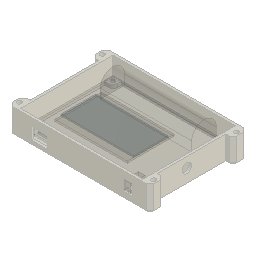
GNSS_Tracker_Enclosure (Autodesk Fusion 360 design; units mm, degrees)
Autodesk Fusion 360 part; units mm, degrees
note: some values were not read from the file. Set by a fixed rule: which sketch regions a step uses.
sketch "Sketch1" plane through (0, 0, 0) normal (0, 0, 1) x (1, 0, 0) in component "GNSS_PCB"
  line L0 (50.5, 37.875) -> (-50.5, 37.875)
  line L1 (-50.5, 37.875) -> (-50.5, -37.875)
  line L2 (-50.5, -37.875) -> (50.5, -37.875)
  line L3 (50.5, -37.875) -> (50.5, 37.875)
  line L4 (50.5, 37.875) -> (-50.5, -37.875) construction
  line L5 (-50.5, 37.875) -> (50.5, -37.875) construction
  line L6 (0, 37.875) -> (0, -37.875) construction
  line L7 (-50.5, 0) -> (50.5, 0) construction
  line L8 (-30.5, 8.425) -> (30.5, 8.425)
  line L9 (30.5, 8.425) -> (30.5, -31.075)
  line L10 (30.5, -31.075) -> (-30.5, -31.075)
  line L11 (-30.5, -31.075) -> (-30.5, 8.425)
  line L12 (-22, 1.425) -> (27.5, 1.425)
  line L13 (27.5, 1.425) -> (27.5, -24.075)
  line L14 (27.5, -24.075) -> (-22, -24.075)
  line L15 (-22, -24.075) -> (-22, 1.425)
  line L16 (-38.5, 35.825) -> (38.5, 35.825)
  line L17 (38.5, 35.825) -> (38.5, 15.175)
  line L18 (38.5, 15.175) -> (-38.5, 15.175)
  line L19 (-38.5, 15.175) -> (-38.5, 35.825)
  line L20 (-33.5, -37.875) -> (-33.5, 37.875) construction
  line L21 (40.5, -37.875) -> (40.5, 37.875) construction
  line L22 (-29, -30.475) -> (-38, -30.475)
  line L23 (-38, -30.475) -> (-38, -37.875)
  line L24 (-38, -37.875) -> (-29, -37.875)
  line L25 (-29, -37.875) -> (-29, -30.475)
  line L26 (-29, -30.475) -> (-38, -37.875) construction
  line L27 (-38, -30.475) -> (-29, -37.875) construction
  line L28 (43.25, -28.875) -> (37.75, -28.875)
  line L29 (37.75, -28.875) -> (37.75, -40.875)
  line L30 (37.75, -40.875) -> (43.25, -40.875)
  line L31 (43.25, -40.875) -> (43.25, -28.875)
  line L32 (43.25, -28.875) -> (37.75, -40.875) construction
  line L33 (37.75, -28.875) -> (43.25, -40.875) construction
  line L34 (50.5, -4) -> (-50.5, -4) construction
  line L35 (-30.5, 3.275) -> (30.5, 3.275)
  line L36 (30.5, 3.275) -> (30.5, -25.925)
  line L37 (30.5, -25.925) -> (-30.5, -25.925)
  line L38 (-30.5, -25.925) -> (-30.5, 3.275)
  point P0 (-48, 35.375)
  point P1 (48, 35.375)
  point P2 (48, -35.375)
  point P3 (-48, -35.375)
  point P4 (-33.5, -34.175)
  point P5 (40.5, -34.875)
  dimension "d6" = 75.75
  dimension "d8" = 101
  dimension "d9" = 2.5
  dimension "d10" = 2.5
  dimension "d19" = 61
  dimension "d20" = 39.5
  dimension "d21" = 30.5
  dimension "d22" = 8.425
  dimension "d23" = 49.5
  dimension "d24" = 25.5
  dimension "d25" = 7
  dimension "d26" = 8.5
  dimension "d30" = 77
  dimension "d31" = 20.65
  dimension "d32" = 38.5
  dimension "d35" = 35.825
  dimension "d38" = 17
  dimension "d39" = 10
  dimension "d43" = 9
  dimension "d44" = 7.4
  dimension "d45" = 7.4
  dimension "d49" = 5.5
  dimension "d50" = 12
  dimension "d51" = 9
  dimension "d74" = 61
  dimension "d75" = 29.2
  dimension "d76" = 5.15
  constraint horizontal L0
  constraint perpendicular L0 L1
  constraint parallel L0 L2
  constraint parallel L1 L3
  constraint coincident L4 origin
  constraint coincident L5 origin
  constraint midpoint L0 L6.start
  constraint midpoint L2 L6.end
  constraint midpoint L1 L7.start
  constraint midpoint L3 L7.end
  constraint symmetric P0 P1 L6
  constraint symmetric P1 P2 L7
  constraint symmetric P0 P3 L7
  constraint horizontal L8
  constraint vertical L9
  constraint horizontal L10
  constraint vertical L11
  constraint horizontal L12
  constraint vertical L13
  constraint horizontal L14
  constraint vertical L15
  constraint horizontal L16
  constraint vertical L17
  constraint horizontal L18
  constraint vertical L19
  constraint coincident L2 L20.start
  constraint coincident L0 L20.end
  constraint perpendicular L0 L20
  constraint coincident L2 L21.start
  constraint coincident L0 L21.end
  constraint perpendicular L0 L21
  constraint horizontal L22
  constraint perpendicular L22 L23
  constraint parallel L22 L24
  constraint parallel L23 L25
  constraint coincident L26 P4
  constraint coincident L27 P4
  constraint coincident L20 P4
  constraint horizontal L28
  constraint perpendicular L28 L29
  constraint parallel L28 L30
  constraint parallel L29 L31
  constraint coincident L32 P5
  constraint coincident L33 P5
  constraint coincident L21 P5
  constraint coincident L3 L34.start
  constraint coincident L1 L34.end
  constraint perpendicular L1 L34
  constraint horizontal L35
  constraint vertical L36
  constraint horizontal L37
  constraint vertical L38
  constraint coincident L11 L35.start
  measures "d6" distance of L0.end L1.end
  measures "d8" distance of L0.start L0.end
  measures "d9" distance of L0 P0
  measures "d10" distance of L1 P0
  measures "d19" distance of L8.start L8.end
  measures "d20" distance of L8.start L10.end
  measures "d21" distance of L6 L11
  measures "d22" distance of L7 L8
  measures "d23" distance of L12.start L12.end
  measures "d24" distance of L12.start L14.end
  measures "d25" distance of L8 L12
  measures "d26" distance of L11 L15
  measures "d30" distance of L16.start L16.end
  measures "d31" distance of L16.start L18.end
  measures "d32" distance of L6 L19
  measures "d35" distance of L7 L16
  measures "d38" distance of L1 L20
  measures "d39" distance of L3 L21
  measures "d43" distance of L23.end L24.end
  measures "d44" distance of L22.end L23.end
  measures "d45" distance of L2 L22
  measures "d49" distance of L29.end L30.end
  measures "d50" distance of L28.end L29.end
  measures "d51" distance of L2 L28
  measures "d74" distance of L35.start L35.end
  measures "d75" distance of L35.start L37.end
  measures "d76" distance of L8 L35
extrude "Extrude1" add sketch "Sketch1" along normal blind 1.6 contours L0 L1 L2 L3 L8 L9 L10 L11 L22 L23 L25 L28 L29 L31 L36 L38 | L2 L28 L29 L31 | L2 L10 L11 L22 L23 L24 L25 | L9 L10 L11 L22 L25 L37 | L10 L11 L22 L25 | L9 L11 L35 L36 L37 L38 | L8 L9 L11 L35 | L12 L13 L14 L15 | L16 L17 L18 L19 makes body 1 in component "GNSS_PCB"
sketch "Sketch2" plane through (0, 0, 1.6) normal (0, 0, 1) x (-1, 0, 0) in component "GNSS_PCB"
  line L0 (50.5, 37.875) -> (-50.5, 37.875)
  line L1 (-50.5, 37.875) -> (-50.5, -37.875)
  line L2 (-50.5, -37.875) -> (50.5, -37.875)
  line L3 (50.5, -37.875) -> (50.5, 37.875)
  line L4 (-37.75, 40.875) -> (-43.25, 40.875)
  line L5 (-37.75, 28.875) -> (-37.75, 40.875)
  line L6 (-43.25, 40.875) -> (-43.25, 28.875)
  line L7 (-40.5, 37.875) -> (-40.5, -37.875)
  line L8 (-38.5, -15.175) -> (38.5, -15.175)
  line L9 (-38.5, -35.825) -> (-38.5, -15.175)
  line L10 (38.5, -15.175) -> (38.5, -35.825)
  line L11 (38.5, -35.825) -> (-38.5, -35.825)
  line L12 (-43.25, 28.875) -> (-37.75, 28.875)
  point P0 (48, 35.375)
  point P1 (48, -35.375)
  point P2 (-48, -35.375)
  point P3 (-48, 35.375)
extrude "Extrude2" add sketch "Sketch2" along normal blind 18.5 contours L8 L9 L10 L11 bodies 1 in component "GNSS_PCB"
extrude "Extrude3" add sketch "Sketch2" along normal blind 7.5 contours L0 L5 L7 L12 | L0 L4 L5 L6 | L0 L6 L7 L12 bodies 1 in component "GNSS_PCB"
fillet "Fillet1" radius 10.325 1 edges at (0, 15.175, 20.1) on bodies 1 in component "GNSS_PCB"
fillet "Fillet2" radius 10.325 1 edges at (0, 35.825, 20.1) on bodies 1 in component "GNSS_PCB"
ref_plane "WorkPlane1" through (0, 0, 3.2) normal (0, 0, 1) x (-1, 0, 0) in component "GNSS_PCB"
sketch "Sketch3" plane through (0, 0, 3.2) normal (0, 0, 1) x (1, 0, 0) in component "GNSS_PCB"
  line L0 (-29, -30.475) -> (-38, -30.475)
  line L1 (-38, -30.475) -> (-38, -37.875)
  line L2 (-29, -37.875) -> (-29, -30.475)
  line L3 (-50.5, -37.875) -> (50.5, -37.875)
extrude "Extrude4" add sketch "Sketch3" along normal blind 1.6 separate body makes body 2 in component "GNSS_PCB"
ref_plane "WorkPlane2" through (0, 0, 12.6) normal (0, 0, 1) x (-1, 0, 0) in component "GNSS_PCB"
sketch "Sketch4" plane through (0, 0, 12.6) normal (0, 0, 1) x (1, 0, 0) in component "GNSS_PCB"
  line L0 (-30.5, 8.425) -> (30.5, 8.425)
  line L1 (-30.5, -31.075) -> (-30.5, 8.425)
  line L2 (30.5, 8.425) -> (30.5, -31.075)
  line L3 (30.5, -31.075) -> (-30.5, -31.075)
extrude "Extrude5" add sketch "Sketch4" along normal blind 1.6 separate body makes body 3 in component "GNSS_PCB"
sketch "Sketch5" plane through (0, 0, 14.2) normal (0, 0, 1) x (-1, 0, 0) in component "GNSS_PCB"
  line L0 (-30.5, 31.075) -> (-30.5, -8.425)
  line L1 (-30.5, -8.425) -> (30.5, -8.425)
  line L2 (30.5, -8.425) -> (30.5, 31.075)
  line L3 (30.5, 31.075) -> (-30.5, 31.075)
sketch "Sketch6" plane through (0, 0, 14.2) normal (0, 0, 1) x (-1, 0, 0) in component "GNSS_PCB"
  line L0 (30.5, -3.275) -> (-30.5, -3.275)
  line L1 (-30.5, 25.925) -> (30.5, 25.925)
  line L2 (30.5, 25.925) -> (30.5, -3.275)
  line L3 (-30.5, -3.275) -> (-30.5, 25.925)
extrude "Extrude6" add sketch "Sketch6" along normal blind 1.3 separate body makes body 4 in component "GNSS_PCB"
sketch "Sketch7" plane through (0, 0, 15.5) normal (0, 0, 1) x (-1, 0, 0) in component "GNSS_PCB"
  line L0 (-30.5, -3.275) -> (30.5, -3.275)
  line L1 (30.5, -3.275) -> (30.5, 25.925)
  line L2 (30.5, 25.925) -> (-30.5, 25.925)
  line L3 (-30.5, 25.925) -> (-30.5, -3.275)
  line L4 (-27.5, 24.075) -> (22, 24.075)
  line L5 (-27.5, -1.425) -> (-27.5, 24.075)
  line L6 (22, 24.075) -> (22, -1.425)
  line L7 (22, -1.425) -> (-27.5, -1.425)
hole "Hole1" at (-48, -35.375, 1.6) at (48, -35.375, 1.6) at (-48, 35.375, 1.6) at (48, 35.375, 1.6) direction (0, 0, -1) diameter 2.1 end through all bodies 1 in component "GNSS_PCB"
ref_plane "WorkPlane1" through (0, 0, -3) normal (0, 0, 1) x (1, 0, 0) in component "GNSS_Enclosure_Bottom"
sketch "Sketch1 (2)" plane through (0, 0, -3) normal (0, 0, 1) x (1, 0, 0) in component "GNSS_Enclosure_Bottom"
  line L0 (-50.5, -37.875) -> (50.5, -37.875)
  line L1 (50.5, -37.875) -> (50.5, 37.875)
  line L2 (50.5, 37.875) -> (-50.5, 37.875)
  line L3 (-50.5, 37.875) -> (-50.5, -37.875)
  line L4 (51.5, -38.875) -> (51.5, 38.875)
  line L5 (51.5, 38.875) -> (-51.5, 38.875)
  line L6 (-51.5, 38.875) -> (-51.5, -38.875)
  line L7 (-51.5, -38.875) -> (51.5, -38.875)
  line L8 (-53.5, -40.875) -> (53.5, -40.875)
  line L9 (53.5, -40.875) -> (53.5, 40.875)
  line L10 (53.5, 40.875) -> (-53.5, 40.875)
  line L11 (-53.5, 40.875) -> (-53.5, -40.875)
  circle A0 centre (-48, 35.375) radius 3.5
  circle A1 centre (48, 35.375) radius 3.5
  circle A2 centre (48, -35.375) radius 3.5
  circle A3 centre (-48, -35.375) radius 3.5
  line L12 (-44.5, 35.375) -> (-44.5, 38.875)
  line L13 (-48, 31.875) -> (-51.5, 31.875)
  line L14 (44.5, 35.375) -> (44.5, 38.875)
  line L15 (48, 31.875) -> (51.5, 31.875)
  line L16 (48, -31.875) -> (51.5, -31.875)
  line L17 (44.5, -35.375) -> (44.5, -38.875)
  line L18 (-48, -31.875) -> (-51.5, -31.875)
  line L19 (-44.5, -35.375) -> (-44.5, -38.875)
  point P0 (48, 35.375)
  point P1 (-48, 35.375)
  point P2 (-48, -35.375)
  point P3 (48, -35.375)
  dimension "d87" = 1
  dimension "d88" = 3
  constraint coincident P1 A0.centre
  constraint tangent L5 A0
  constraint coincident P0 A1.centre
  constraint tangent L5 A1
  constraint coincident P3 A2.centre
  constraint tangent L4 A2
  constraint coincident P2 A3.centre
  constraint tangent L7 A3
  constraint coincident A0 L12.start
  constraint coincident L5 L12.end
  constraint tangent A0 L12
  constraint perpendicular L5 L12
  constraint coincident A0 L13.start
  constraint coincident L6 L13.end
  constraint tangent A0 L13
  constraint perpendicular L6 L13
  constraint coincident A1 L14.start
  constraint coincident L5 L14.end
  constraint tangent A1 L14
  constraint perpendicular L5 L14
  constraint coincident A1 L15.start
  constraint coincident L4 L15.end
  constraint tangent A1 L15
  constraint perpendicular L4 L15
  constraint coincident A2 L16.start
  constraint coincident L4 L16.end
  constraint tangent A2 L16
  constraint perpendicular L4 L16
  constraint coincident A2 L17.start
  constraint coincident L7 L17.end
  constraint tangent A2 L17
  constraint perpendicular L7 L17
  constraint coincident A3 L18.start
  constraint coincident L6 L18.end
  constraint tangent A3 L18
  constraint perpendicular L6 L18
  constraint coincident A3 L19.start
  constraint coincident L7 L19.end
  constraint tangent A3 L19
  constraint perpendicular L7 L19
extrude "Extrude1'" add sketch "Sketch1 (2)" against normal blind 2 separate body contours L0 L3 A3 | L0 L3 L6 L7 A3 | L0 L3 A3 | L0 A3 | L3 A3 | L0 A3 L19 | L0 L7 A3 L19 | L3 L6 A3 L18 | L3 A3 L18 | L0 L1 L2 L3 A0 A1 A2 A3 L12 L13 L14 L15 L16 L17 L18 L19 | L0 L7 L17 L19 | L3 L6 L13 L18 | L0 A2 L17 | L0 L7 A2 L17 | L3 L6 A0 L13 | L3 A0 L13 | L0 L1 A2 | L0 A2 | L0 L1 L4 L7 A2 | L3 A0 | L2 L3 A0 | L2 L3 L5 L6 A0 | L0 L1 A2 | L1 A2 L16 | L2 L3 A0 | L2 A0 L12 | L1 A2 | L1 L4 A2 L16 | L1 L4 L15 L16 | L2 A0 | L2 L5 A0 L12 | L2 L5 L12 L14 | L1 A1 L15 | L1 L4 A1 L15 | L2 L5 A1 L14 | L2 A1 L14 | L1 L2 A1 | L1 A1 | L2 A1 | L1 L2 A1 | L1 L2 L4 L5 A1 | L8 L9 L10 L11 makes body 5 in component "GNSS_Enclosure_Bottom"
extrude "Extrude2'" add sketch "Sketch1 (2)" along normal up to surface (18.5 mm away) bodies 5 in component "GNSS_Enclosure_Bottom"
extrude "Extrude3'" add sketch "Sketch1 (2)" along normal blind 3 contours L0 L3 A3 | L0 L3 L6 L7 A3 | L0 L3 A3 | L0 A3 | L3 A3 | L0 A3 L19 | L0 L7 A3 L19 | L3 L6 A3 L18 | L3 A3 L18 | L0 A2 L17 | L0 L7 A2 L17 | L3 L6 A0 L13 | L3 A0 L13 | L0 L1 A2 | L0 A2 | L0 L1 L4 L7 A2 | L3 A0 | L2 L3 A0 | L2 L3 L5 L6 A0 | L1 A2 L16 | L2 A0 L12 | L1 A2 | L1 L4 A2 L16 | L2 A0 | L2 L5 A0 L12 | L1 A1 L15 | L1 L4 A1 L15 | L2 L5 A1 L14 | L2 A1 L14 | L1 L2 A1 | L1 A1 | L2 A1 | L1 L2 L4 L5 A1 picked at (48.5119, -35.209) picked at (-48.8502, 36.2083) picked at (47.5153, 35.9804) bodies 5 in component "GNSS_Enclosure_Bottom"
sketch "Sketch2 (2)" plane through (0, 0, 0) normal (0, 0, 1) x (-1, 0, 0) in component "GNSS_Enclosure_Bottom"
  line L0 (-50.5, -37.875) -> (-50.5, -37.8245)
  arc A0 (-50.5, -37.8245) -> (-50.4495, -37.875) centre (-48, -35.375) ccw
  line L1 (-50.4495, -37.875) -> (-50.5, -37.875)
  arc A1 (-44.5, -35.375) -> (-48, -31.875) centre (-48, -35.375) ccw
  line L2 (-48, -31.875) -> (-51.5, -31.875)
  line L3 (-51.5, -31.875) -> (-51.5, -38.875)
  line L4 (-51.5, -38.875) -> (-44.5, -38.875)
  line L5 (-44.5, -38.875) -> (-44.5, -35.375)
  point P0 (-48, 35.375)
  point P1 (48, 35.375)
  point P2 (48, -35.375)
  point P3 (-48, -35.375)
hole "Hole1'" at (48, -35.375, 0) at (-48, -35.375, 0) at (48, 35.375, 0) at (-48, 35.375, 0) direction (0, 0, -1) diameter 3.4 depth 3 tip angle 180 bodies 5 in component "GNSS_Enclosure_Bottom"
sketch "Sketch3 (2)" plane through (0, -40.875, 0) normal (0, -1, 0) x (1, 0, 0) in component "GNSS_Enclosure_Bottom"
  line L0 (-53.5, 15.5) -> (-53.5, -5)
  line L1 (-53.5, -5) -> (53.5, -5)
  line L2 (53.5, -5) -> (53.5, 15.5)
  line L3 (53.5, 15.5) -> (-53.5, 15.5)
  line L4 (-38, 3.2) -> (-29, 3.2)
  line L5 (-29, 3.2) -> (-29, 4.8)
  line L6 (-29, 4.8) -> (-38, 4.8)
  line L7 (-38, 4.8) -> (-38, 3.2)
  line L8 (37.75, 1.6) -> (43.25, 1.6)
  line L9 (43.25, 1.6) -> (43.25, 9.1)
  line L10 (43.25, 9.1) -> (37.75, 9.1)
  line L11 (37.75, 9.1) -> (37.75, 1.6)
  line L12 (36.75, 10.1) -> (36.75, 0.6)
  line L13 (36.75, 0.6) -> (44.25, 0.6)
  line L14 (44.25, 0.6) -> (44.25, 10.1)
  line L15 (44.25, 10.1) -> (36.75, 10.1)
  line L16 (-33.5, 4.8) -> (-33.5, 3.2) construction
  line L17 (-38, 4) -> (-29, 4) construction
  line L18 (-26.5, 9) -> (-40.5, 9)
  line L19 (-40.5, 9) -> (-40.5, -1)
  line L20 (-40.5, -1) -> (-26.5, -1)
  line L21 (-26.5, -1) -> (-26.5, 9)
  line L22 (-26.5, 9) -> (-40.5, -1) construction
  line L23 (-40.5, 9) -> (-26.5, -1) construction
  point P0 (-33.5, 4)
  dimension "d102" = 1
  dimension "d107" = 14
  dimension "d108" = 10
  constraint midpoint L6 L16.start
  constraint midpoint L4 L16.end
  constraint midpoint L7 L17.start
  constraint midpoint L5 L17.end
  constraint horizontal L18
  constraint perpendicular L18 L19
  constraint parallel L18 L20
  constraint parallel L19 L21
  constraint coincident L22 P0
  constraint coincident L23 P0
  constraint midpoint L17 P0
  measures "d107" distance of L19.end L20.end
  measures "d108" distance of L18.end L19.end
extrude "Extrude4'" cut sketch "Sketch3 (2)" against normal up to surface (2 mm away) contours L8 L9 L10 L11 | L12 L13 L14 L15 bodies 5 in component "GNSS_Enclosure_Bottom"
extrude "Extrude5'" cut sketch "Sketch3 (2)" against normal up to surface (2 mm away) contours L4 L5 L6 L7 | L18 L19 L20 L21 bodies 5 in component "GNSS_Enclosure_Bottom"
sketch "Sketch1 (3)" plane through (0, 0, 15.5) normal (0, 0, 1) x (-1, 0, 0) in component "GNSS_Enclosure_Top"
  line L0 (-51.5, -38.875) -> (-51.5, 38.875)
  line L1 (-51.5, 38.875) -> (51.5, 38.875)
  line L2 (51.5, 38.875) -> (51.5, -38.875)
  line L3 (51.5, -38.875) -> (-51.5, -38.875)
  line L4 (-53.5, -40.875) -> (53.5, -40.875)
  line L5 (53.5, -40.875) -> (53.5, 40.875)
  line L6 (53.5, 40.875) -> (-53.5, 40.875)
  line L7 (-53.5, 40.875) -> (-53.5, -40.875)
  line L8 (-38.5, -35.825) -> (-38.5, -15.175)
  line L9 (38.5, -35.825) -> (-38.5, -35.825)
  line L10 (-38.5, -15.175) -> (38.5, -15.175)
  line L11 (38.5, -15.175) -> (38.5, -35.825)
  line L12 (53.5, -40.875) -> (-53.5, -40.875)
  line L13 (53.5, 40.875) -> (53.5, -40.875)
  line L14 (-53.5, -40.875) -> (-53.5, 40.875)
  line L15 (-53.5, 40.875) -> (53.5, 40.875)
  line L16 (53.5, -10.125) -> (-53.5, -10.125)
  line L17 (-51.5, 38.875) -> (-51.5, -38.875)
  line L18 (-51.5, -38.875) -> (51.5, -38.875)
  line L19 (51.5, -38.875) -> (51.5, 38.875)
  dimension "d111" = 5.05
  dimension "d112" = 5.05
  constraint coincident L13 L16.start
  constraint coincident L14 L16.end
  constraint perpendicular L14 L16
  measures "d111" distance of L4 L9
  measures "d112" distance of L10 L16
extrude "Extrude1''" add sketch "Sketch1 (3)" along normal blind 2 separate body contours L0 L2 L3 L4 L5 L7 L12 L13 L14 L16 L17 L18 L19 | L0 L1 L2 L5 L6 L7 L13 L14 L15 L16 L17 L19 | L0 L1 L2 L16 L17 L19 makes body 6 in component "GNSS_Enclosure_Top"
sketch "Sketch2 (3)" plane through (0, 0, 17.5) normal (0, 0, 1) x (-1, 0, 0) in component "GNSS_Enclosure_Top"
  line L0 (51.5, -10.125) -> (51.5, -38.875)
  line L1 (51.5, -38.875) -> (-51.5, -38.875)
  line L2 (-51.5, -38.875) -> (-51.5, -10.125)
  line L3 (-51.5, -10.125) -> (51.5, -10.125)
  line L4 (-53.5, 40.875) -> (-53.5, -40.875)
  line L5 (-53.5, -40.875) -> (53.5, -40.875)
  line L6 (53.5, -40.875) -> (53.5, 40.875)
  line L7 (53.5, 40.875) -> (-53.5, 40.875)
  line L8 (-53.5, -8.125) -> (53.5, -8.125)
  dimension "d115" = 2
  constraint coincident L4 L8.start
  constraint coincident L6 L8.end
  constraint perpendicular L6 L8
  measures "d115" distance of L3 L8
sketch "Sketch3 (3)" plane through (53.5, 0, 0) normal (1, 0, 0) x (0, 1, 0) in component "GNSS_Enclosure_Top"
  line L0 (-40.875, 15.5) -> (40.875, 15.5)
  line L1 (40.875, 15.5) -> (40.875, 17.5)
  line L2 (40.875, 17.5) -> (-40.875, 17.5)
  line L3 (-40.875, 17.5) -> (-40.875, 15.5)
  arc A0 (35.825, 9.775) -> (15.175, 9.775) centre (25.5, 9.775) ccw
  line L4 (25.5, 20.1) -> (40.875, 20.1) construction
  line L5 (40.875, 20.1) -> (40.875, 17.5) construction
  line L6 (25.5, 22.1) -> (42.875, 22.1) construction
  line L7 (42.875, 22.1) -> (42.875, 17.5) construction
  constraint midpoint A0 L4.start
  constraint tangent A0 L4
  constraint perpendicular L1 L4
  constraint coincident L1.end L2.start
  constraint perpendicular L2 L5
extrude "Extrude2''" add sketch "Sketch2 (3)" along normal up to surface (4.6 mm away) contours L4 L5 L6 L8 bodies 6 in component "GNSS_Enclosure_Top"
sketch "Sketch4 (2)" plane through (0, 0, 22.1) normal (0, 0, 1) x (-1, 0, 0) in component "GNSS_Enclosure_Top"
  line L0 (51.5, -38.875) -> (-51.5, -38.875)
  line L1 (-51.5, -38.875) -> (-51.5, -10.125)
  line L2 (-51.5, -10.125) -> (51.5, -10.125)
  line L3 (51.5, -10.125) -> (51.5, -38.875)
  line L4 (-53.5, -8.125) -> (-53.5, -40.875)
  line L5 (-53.5, -40.875) -> (53.5, -40.875)
  line L6 (53.5, -40.875) -> (53.5, -8.125)
  line L7 (53.5, -8.125) -> (-53.5, -8.125)
extrude "Extrude3''" add sketch "Sketch4 (2)" along normal blind 2 contours L0 L1 L2 L3 | L4 L5 L6 L7 bodies 6 in component "GNSS_Enclosure_Top"
sketch "Sketch4 (3)" plane through (53.5, 0, 0) normal (1, 0, 0) x (0, 1, 0) in component "GNSS_Enclosure_Bottom"
  line L0 (-40.875, 15.5) -> (-40.875, -5)
  line L1 (-40.875, -5) -> (40.875, -5)
  line L2 (40.875, -5) -> (40.875, 15.5)
  line L3 (40.875, 15.5) -> (-40.875, 15.5)
  line L4 (-4, 0) -> (-4, 15.5) construction
  point P0 (-4, 0)
  point P1 (-4, 7.1)
  dimension "d124" = 7.1
  constraint coincident P0 L4.start
  constraint coincident L3 L4.end
  constraint perpendicular L3 L4
  constraint coincident L4 P1
  measures "d124" distance of P0 P1
hole "Hole2" at (53.5, -4, 7.1) direction (-1, 0, 0) diameter 8 depth 2 tip angle 180 bodies 5 in component "GNSS_Enclosure_Bottom"
sketch "Sketch5 (2)" plane through (0, 0, -5) normal (0, 0, -1) x (1, 0, 0) in component "GNSS_Enclosure_Bottom"
  line L0 (-53.5, 40.875) -> (-53.5, -40.875)
  line L1 (-53.5, -40.875) -> (53.5, -40.875)
  line L2 (53.5, -40.875) -> (53.5, 40.875)
  line L3 (53.5, 40.875) -> (-53.5, 40.875)
  line L4 (-53.5, 40.875) -> (-53.5, -40.875)
  line L5 (53.5, -40.875) -> (53.5, 40.875)
  line L6 (59.5, -40.875) -> (59.5, 40.875) construction
  line L7 (-59.5, 40.875) -> (-59.5, -40.875) construction
  line L8 (59.5, -40.875) -> (53.5, -40.875) construction
  line L9 (59.5, 40.875) -> (53.5, 40.875) construction
  line L10 (-59.5, -40.875) -> (-53.5, -40.875) construction
  line L11 (-59.5, 40.875) -> (-53.5, 40.875) construction
  line L12 (59.5, -28.875) -> (53.5, -28.875) construction
  line L13 (56.5, -40.875) -> (56.5, -28.875) construction
  line L14 (53.5, -40.875) -> (59.5, -40.875)
  line L15 (59.5, -28.875) -> (59.5, -40.875)
  line L16 (59.5, -28.875) -> (53.5, -28.875)
  line L17 (59.5, 28.875) -> (53.5, 28.875)
  line L18 (59.5, 28.875) -> (59.5, 40.875)
  line L19 (59.5, 40.875) -> (53.5, 40.875)
  line L20 (-59.5, -28.875) -> (-53.5, -28.875)
  line L21 (-59.5, 28.875) -> (-53.5, 28.875)
  line L22 (-53.5, -40.875) -> (-59.5, -40.875)
  line L23 (-59.5, -28.875) -> (-59.5, -40.875)
  line L24 (-59.5, 28.875) -> (-59.5, 40.875)
  line L25 (-59.5, 40.875) -> (-53.5, 40.875)
  line L26 (56.5, 28.875) -> (56.5, 40.875) construction
  line L27 (59.5, 34.875) -> (53.5, 34.875) construction
  line L28 (-56.5, -40.875) -> (-56.5, -28.875) construction
  line L29 (-56.5, 28.875) -> (-56.5, 40.875) construction
  point P0 (56.5, -34.875)
  point P1 (-56.5, -34.875)
  point P2 (-56.5, 34.875)
  point P3 (56.5, 34.875)
  dimension "d129" = 6
  dimension "d130" = 6
  dimension "d131" = 12
  dimension "d132" = 12
  dimension "d133" = 12
  dimension "d134" = 12
  constraint coincident L1.end L2.start
  constraint perpendicular L5 L8
  constraint coincident L2.end L3.start
  constraint perpendicular L5 L9
  constraint coincident L0.end L1.start
  constraint perpendicular L4 L10
  constraint coincident L0.start L3.end
  constraint perpendicular L4 L11
  constraint coincident L6 L12.start
  constraint coincident L2 L12.end
  constraint perpendicular L2 L12
  constraint midpoint L8 L13.start
  constraint midpoint L12 L13.end
  constraint midpoint L13 P0
  constraint coincident L6 L17.start
  constraint coincident L5 L17.end
  constraint perpendicular L5 L17
  constraint coincident L7 L20.start
  constraint coincident L0 L20.end
  constraint perpendicular L0 L20
  constraint coincident L7 L21.start
  constraint coincident L4 L21.end
  constraint perpendicular L4 L21
  constraint midpoint L17 L26.start
  constraint midpoint L9 L26.end
  constraint midpoint L18 L27.start
  constraint coincident L5 L27.end
  constraint perpendicular L5 L27
  constraint midpoint L10 L28.start
  constraint midpoint L20 L28.end
  constraint midpoint L21 L29.start
  constraint midpoint L25 L29.end
  constraint midpoint L28 P1
  constraint midpoint L29 P2
  constraint midpoint L26 P3
  measures "d131" distance of L8 L12
  measures "d132" distance of L9 L17
  measures "d133" distance of L10 L20
  measures "d134" distance of L11 L21
extrude "Extrude6'" add sketch "Sketch5 (2)" against normal up to surface (20.5 mm away) contours L0 L4 L21 L24 L25 | L2 L5 L17 L18 L19 | L0 L4 L20 L22 L23 | L2 L5 L14 L15 L16 bodies 5 in component "GNSS_Enclosure_Bottom"
chamfer "Chamfer1" distance 3 angle 45 8 edges at (59.5, -40.875, 5.25) (59.5, 40.875, 5.25) (59.5, 28.875, 5.25) (59.5, -28.875, 5.25) (-59.5, -40.875, 5.25) (-59.5, -28.875, 5.25) (-59.5, 28.875, 5.25) (-59.5, 40.875, 5.25) on bodies 5 in component "GNSS_Enclosure_Bottom"
sketch "Sketch6 (2)" plane through (0, 0, 15.5) normal (0, 0, 1) x (-1, 0, 0) in component "GNSS_Enclosure_Bottom"
  line L0 (-51.5, -38.875) -> (-51.5, 38.875)
  line L1 (-51.5, 38.875) -> (51.5, 38.875)
  line L2 (51.5, 38.875) -> (51.5, -38.875)
  line L3 (51.5, -38.875) -> (-51.5, -38.875)
  line L4 (56.5, -40.875) -> (59.5, -37.875)
  line L5 (59.5, -37.875) -> (59.5, -31.875)
  line L6 (59.5, -31.875) -> (56.5, -28.875)
  line L7 (56.5, -28.875) -> (53.5, -28.875)
  line L8 (53.5, -28.875) -> (53.5, 28.875)
  line L9 (53.5, 28.875) -> (56.5, 28.875)
  line L10 (56.5, 28.875) -> (59.5, 31.875)
  line L11 (59.5, 31.875) -> (59.5, 37.875)
  line L12 (59.5, 37.875) -> (56.5, 40.875)
  line L13 (56.5, 40.875) -> (-56.5, 40.875)
  line L14 (-56.5, 40.875) -> (-59.5, 37.875)
  line L15 (-59.5, 37.875) -> (-59.5, 31.875)
  line L16 (-59.5, 31.875) -> (-56.5, 28.875)
  line L17 (-56.5, 28.875) -> (-53.5, 28.875)
  line L18 (-53.5, 28.875) -> (-53.5, -28.875)
  line L19 (-53.5, -28.875) -> (-56.5, -28.875)
  line L20 (-56.5, -28.875) -> (-59.5, -31.875)
  line L21 (-59.5, -31.875) -> (-59.5, -37.875)
  line L22 (-59.5, -37.875) -> (-56.5, -40.875)
  line L23 (-56.5, -40.875) -> (56.5, -40.875)
  line L24 (-53.5, -28.875) -> (-53.5, -40.875)
  line L25 (53.5, -28.875) -> (53.5, -40.875)
  point P0 (-56.5, 34.875)
  point P1 (-56.5, -34.875)
  point P2 (56.5, -34.875)
  point P3 (56.5, 34.875)
  point P4 (-53.5, -40.875)
  point P5 (53.5, -40.875)
  constraint coincident L18.end L19.start
  constraint coincident P4 L24.end
  constraint coincident L7.end L8.start
  constraint coincident P5 L25.end
hole "Hole3" at (-56.5, -34.875, 15.5) at (-56.5, 34.875, 15.5) at (56.5, -34.875, 15.5) at (56.5, 34.875, 15.5) direction (0, 0, -1) diameter 3.4 depth 3 tip angle 180 bodies 5 in component "GNSS_Enclosure_Bottom"
chamfer "Chamfer2" distance 0.2 distance2 3 8 edges at (-58.085, 35.4897, 15.5) (54.915, 35.4897, 15.5) (-49.585, 35.9897, 0) (-58.085, -34.2603, 15.5) (54.915, -34.2603, 15.5) (46.415, 35.9897, 0) (46.415, -34.7603, 0) (-49.585, -34.7603, 0) measured on face at (54.557, -38.703, 15.5) measured on face at (54.557, -38.703, 15.5) measured on face at (-45.1759, 36.825, 0) measured on face at (54.557, -38.703, 15.5) measured on face at (54.557, -38.703, 15.5) measured on face at (45.1759, 36.825, 0) measured on face at (45.1759, -36.825, 0) measured on face at (-50.8984, -35.3327, 0) on bodies 5 in component "GNSS_Enclosure_Bottom"
sketch "Sketch5 (3)" plane through (0, 0, 15.5) normal (0, 0, -1) x (1, 0, 0) in component "GNSS_Enclosure_Top"
  line L0 (-51.5, -38.875) -> (-51.5, -10.125)
  line L1 (-51.5, -10.125) -> (51.5, -10.125)
  line L2 (51.5, -10.125) -> (51.5, -38.875)
  line L3 (51.5, -38.875) -> (-51.5, -38.875)
  line L4 (53.5, -40.875) -> (53.5, 40.875)
  line L5 (53.5, 40.875) -> (-53.5, 40.875)
  line L6 (-53.5, 40.875) -> (-53.5, -40.875)
  line L7 (-53.5, -40.875) -> (53.5, -40.875)
  circle A0 centre (-56.5, 34.875) radius 1.9
  circle A1 centre (-56.5, -34.875) radius 1.9
  line L8 (51.5, -38.875) -> (51.5, 38.875)
  line L9 (51.5, 38.875) -> (-51.5, 38.875)
  line L10 (-51.5, 38.875) -> (-51.5, -38.875)
  line L11 (-51.5, -38.875) -> (51.5, -38.875)
  line L12 (-56.5, -40.875) -> (-59.5, -37.875)
  line L13 (-59.5, -37.875) -> (-59.5, -31.875)
  line L14 (-59.5, -31.875) -> (-56.5, -28.875)
  line L15 (-56.5, -28.875) -> (-53.5, -28.875)
  line L16 (-53.5, -28.875) -> (-53.5, 28.875)
  line L17 (-53.5, 28.875) -> (-56.5, 28.875)
  line L18 (-56.5, 28.875) -> (-59.5, 31.875)
  line L19 (-59.5, 31.875) -> (-59.5, 37.875)
  line L20 (-59.5, 37.875) -> (-56.5, 40.875)
  line L21 (-56.5, 40.875) -> (56.5, 40.875)
  line L22 (56.5, 40.875) -> (59.5, 37.875)
  line L23 (59.5, 37.875) -> (59.5, 31.875)
  line L24 (59.5, 31.875) -> (56.5, 28.875)
  line L25 (56.5, 28.875) -> (53.5, 28.875)
  line L26 (53.5, 28.875) -> (53.5, -28.875)
  line L27 (53.5, -28.875) -> (56.5, -28.875)
  line L28 (56.5, -28.875) -> (59.5, -31.875)
  line L29 (59.5, -31.875) -> (59.5, -37.875)
  line L30 (59.5, -37.875) -> (56.5, -40.875)
  line L31 (56.5, -40.875) -> (-56.5, -40.875)
  circle A2 centre (56.5, -34.875) radius 1.9
  circle A3 centre (56.5, 34.875) radius 1.9
extrude "Extrude4''" add sketch "Sketch5 (3)" against normal up to surface (2 mm away) contours L4 L21 L22 L23 L24 L25 | L6 L17 L18 L19 L20 L21 | A0 | A3 bodies 6 in component "GNSS_Enclosure_Top"
extrude "Extrude5''" add sketch "Sketch6 (2)" along normal up to surface (8.6 mm away) contours L4 L5 L6 L7 L23 L25 | L19 L20 L21 L22 L23 L24 bodies 6 in component "GNSS_Enclosure_Top"
sketch "Sketch6 (3)" plane through (0, 0, 15.5) normal (0, 0, 1) x (1, 0, 0) in component "GNSS_Enclosure_Top"
sketch "Sketch7 (2)" plane through (0, 0, 17.5) normal (0, 0, 1) x (-1, 0, 0) in component "GNSS_Enclosure_Top"
  line L0 (-53.5, -8.125) -> (53.5, -8.125)
  line L1 (53.5, -8.125) -> (53.5, 28.875)
  line L2 (53.5, 28.875) -> (56.5, 28.875)
  line L3 (56.5, 28.875) -> (59.5, 31.875)
  line L4 (59.5, 31.875) -> (59.5, 37.875)
  line L5 (59.5, 37.875) -> (56.5, 40.875)
  line L6 (56.5, 40.875) -> (-56.5, 40.875)
  line L7 (-56.5, 40.875) -> (-59.5, 37.875)
  line L8 (-59.5, 37.875) -> (-59.5, 31.875)
  line L9 (-59.5, 31.875) -> (-56.5, 28.875)
  line L10 (-56.5, 28.875) -> (-53.5, 28.875)
  line L11 (-53.5, 28.875) -> (-53.5, -8.125)
  point P0 (56.5, 34.875)
  point P1 (-56.5, 34.875)
sketch "Sketch8" plane through (0, 0, 24.1) normal (0, 0, 1) x (-1, 0, 0) in component "GNSS_Enclosure_Top"
  line L0 (53.5, -8.125) -> (-53.5, -8.125)
  line L1 (-53.5, -8.125) -> (-53.5, -28.875)
  line L2 (-53.5, -28.875) -> (-56.5, -28.875)
  line L3 (-56.5, -28.875) -> (-59.5, -31.875)
  line L4 (-59.5, -31.875) -> (-59.5, -37.875)
  line L5 (-59.5, -37.875) -> (-56.5, -40.875)
  line L6 (-56.5, -40.875) -> (56.5, -40.875)
  line L7 (56.5, -40.875) -> (59.5, -37.875)
  line L8 (59.5, -37.875) -> (59.5, -31.875)
  line L9 (59.5, -31.875) -> (56.5, -28.875)
  line L10 (56.5, -28.875) -> (53.5, -28.875)
  line L11 (53.5, -28.875) -> (53.5, -8.125)
  point P0 (56.5, -34.875)
  point P1 (-56.5, -34.875)
hole "Hole1''" at (-56.5, 34.875, 24.1) at (56.5, 34.875, 24.1) direction (0, 0, -1) diameter 2.3 depth 8.6 tip angle 180 counterbore diameter 4 counterbore depth 2 bodies 6 in component "GNSS_Enclosure_Top"
hole "Hole2'" at (-56.5, -34.875, 17.5) at (56.5, -34.875, 17.5) direction (0, 0, -1) diameter 2.3 depth 2 tip angle 180 counterbore diameter 4 counterbore depth 1 bodies 6 in component "GNSS_Enclosure_Top"
sketch "Sketch9" plane through (0, 0, 17.5) normal (0, 0, 1) x (-1, 0, 0) in component "GNSS_Enclosure_Top"
  circle A0 centre (56.5, 34.875) radius 2
  circle A1 centre (-56.5, 34.875) radius 2
  line L0 (-53.5, -8.125) -> (53.5, -8.125)
  line L1 (53.5, -8.125) -> (53.5, 28.875)
  line L2 (53.5, 28.875) -> (56.5, 28.875)
  line L3 (56.5, 28.875) -> (59.5, 31.875)
  line L4 (59.5, 31.875) -> (59.5, 37.875)
  line L5 (59.5, 37.875) -> (56.5, 40.875)
  line L6 (56.5, 40.875) -> (-56.5, 40.875)
  line L7 (-56.5, 40.875) -> (-59.5, 37.875)
  line L8 (-59.5, 37.875) -> (-59.5, 31.875)
  line L9 (-59.5, 31.875) -> (-56.5, 28.875)
  line L10 (-56.5, 28.875) -> (-53.5, 28.875)
  line L11 (-53.5, 28.875) -> (-53.5, -8.125)
  line L12 (22, -1.425) -> (-27.5, -1.425)
  line L13 (22, 24.075) -> (22, -1.425)
  line L14 (-27.5, 24.075) -> (22, 24.075)
  line L15 (-27.5, -1.425) -> (-27.5, 24.075)
extrude "Extrude6''" cut sketch "Sketch9" against normal up to surface (2 mm away) contours L12 L13 L14 L15 bodies 6 in component "GNSS_Enclosure_Top"
chamfer "Chamfer1'" distance 2 angle 45 4 edges at (2.75, 1.425, 17.5) (27.5, -11.325, 17.5) (2.75, -24.075, 17.5) (-22, -11.325, 17.5) on bodies 6 in component "GNSS_Enclosure_Top"
chamfer "Chamfer2'" distance 1 angle 45 25 edges at (59.5, -34.875, 17.5) (58, -30.375, 17.5) (55, -28.875, 17.5) (53.5, -10.375, 17.5) (58, -39.375, 17.5) (0, -40.875, 17.5) (-58, -39.375, 17.5) (-59.5, -34.875, 17.5) (-58, -30.375, 17.5) (-55, -28.875, 17.5) (-53.5, -10.375, 17.5) (-53.5, 8.125, 20.8) (-53.5, 18.5, 24.1) (0, 8.125, 24.1) (-55, 28.875, 24.1) (-58, 30.375, 24.1) (-59.5, 34.875, 24.1) (-58, 39.375, 24.1) (0, 40.875, 24.1) (58, 39.375, 24.1) (59.5, 34.875, 24.1) (58, 30.375, 24.1) (55, 28.875, 24.1) (53.5, 18.5, 24.1) (53.5, 8.125, 20.8) on bodies 6 in component "GNSS_Enclosure_Top"
chamfer "Chamfer3" distance 1 angle 45 20 edges at (0, -40.875, -5) (-58, -39.375, -5) (-59.5, -34.875, -5) (-58, -30.375, -5) (-55, -28.875, -5) (-53.5, 0, -5) (58, -39.375, -5) (59.5, -34.875, -5) (58, -30.375, -5) (55, -28.875, -5) (53.5, 0, -5) (55, 28.875, -5) (58, 30.375, -5) (59.5, 34.875, -5) (58, 39.375, -5) (0, 40.875, -5) (-58, 39.375, -5) (-59.5, 34.875, -5) (-58, 30.375, -5) (-55, 28.875, -5) on bodies 5 in component "GNSS_Enclosure_Bottom"
component "GNSS_PCB" placed x (1, 0, 0) y (0, 1, 0) z (0, 0, 1) at (0, 0, 0)
component "GNSS_Enclosure_Bottom" placed x (1, 0, 0) y (0, 1, 0) z (0, 0, 1) at (0, 0, 0)
component "GNSS_Enclosure_Top" placed x (1, 0, 0) y (0, 1, 0) z (0, 0, 1) at (0, 0, 0)
equation "PCB_X_Size = 100 mm"
equation "PCB_Y_Size = 75 mm"
equation "PCB_Bolt_Inset = 2.5 mm"
equation "PCB_Z_Size = 1.6 mm"
equation "d6 = PCB_Y_Size + ( PCB_Y_Size * PCB_Shrinkage_Percent )"
equation "PCB_Shrinkage_Percent = 0.01"
equation "d8 = PCB_X_Size + ( PCB_X_Size * PCB_Shrinkage_Percent )"
equation "d9 = PCB_Bolt_Inset"
equation "d10 = PCB_Bolt_Inset"
equation "Screen_PCB_X_Size = 61 mm"
equation "Screen_PCB_Y_Size = 39.5 mm"
equation "Screen_DisplayArea_X_Size = 49.5 mm"
equation "Screen_DisplayArea_Y_Size = 25.5 mm"
equation "Screen_DisplayArea_X_Offset = 8.5 mm"
equation "Screen_DisplayArea_Y_Offset = 7.5 mm"
equation "Screen_Center_X_Offset = 0 mm"
equation "Screen_Center_Y_Offset = -11.325 mm"
equation "d19 = Screen_PCB_X_Size"
equation "d20 = Screen_PCB_Y_Size"
equation "d21 = ( Screen_PCB_X_Size / 2 ) + Screen_Center_X_Offset"
equation "d22 = ( Screen_PCB_Y_Size / 2 ) + Screen_Center_Y_Offset"
equation "d23 = Screen_DisplayArea_X_Size"
equation "d24 = Screen_DisplayArea_Y_Size"
equation "d25 = ( Screen_PCB_Y_Size - Screen_DisplayArea_Y_Size ) / 2"
equation "d26 = Screen_DisplayArea_X_Offset"
equation "BatteryHolder_X_Size = 77 mm"
equation "BatteryHolder_Y_Size = 20.65 mm"
equation "BatteryHolder_Z_Size = 18.5 mm"
equation "d30 = BatteryHolder_X_Size"
equation "d31 = BatteryHolder_Y_Size"
equation "d32 = ( BatteryHolder_X_Size / 2 ) + BatteryHolder_Center_X_Offset"
equation "BatteryHolder_Center_X_Offset = 0 mm"
equation "BatteryHolder_Center_Y_Offset = 25.5 mm"
equation "d35 = ( BatteryHolder_Y_Size / 2 ) + BatteryHolder_Center_Y_Offset"
equation "USB_X_Center_Offset = 17 mm"
equation "SolarInput_X_CenterOffset = 10 mm"
equation "d38 = USB_X_Center_Offset"
equation "d39 = SolarInput_X_CenterOffset"
equation "USB_Jack_X_Size = 9 mm"
equation "USB_Jack_Z_Size = 3.2 mm"
equation "USB_Jack_Y_Size = 7.4 mm"
equation "d43 = USB_Jack_X_Size"
equation "d44 = USB_Jack_Y_Size"
equation "d45 = USB_Jack_Y_Size"
equation "SolarInput_X_Size = 5.5 mm"
equation "SolarInput_Y_Size = 12 mm"
equation "SolarInput_Z_Size = 7.5 mm"
equation "d49 = SolarInput_X_Size"
equation "d50 = SolarInput_Y_Size"
equation "d51 = SolarInput_Y_Size - SolarInput_EdgeOverhang"
equation "SolarInput_EdgeOverhang = 3 mm"
equation "Antenna_PCB_Center_Offset = -4 mm"
equation "d54 = -Antenna_PCB_Center_Offset"
equation "d55 = PCB_Z_Size"
equation "d57 = BatteryHolder_Z_Size"
equation "d59 = SolarInput_Z_Size"
equation "d62 = BatteryHolder_Y_Size / 2"
equation "d64 = BatteryHolder_Y_Size / 2"
equation "d65 = PCB_Z_Size"
equation "d66 = PCB_Z_Size"
equation "Screen_Z_Offset = 11 mm"
equation "d69 = Screen_Z_Offset"
equation "d70 = PCB_Z_Size"
equation "Screen_Display_Z_Size = 1.3 mm"
equation "Screen_Y_Size = 29.2 mm"
equation "d74 = Screen_PCB_X_Size"
equation "d75 = Screen_Y_Size"
equation "d76 = ( Screen_PCB_Y_Size - Screen_Y_Size ) / 2"
equation "d77 = Screen_Display_Z_Size"
equation "d80 = PCB_Bolt_Hole_Diameter"
equation "PCB_Bolt_Hole_Diameter = 2.1 mm"
equation "Enclosure_Wall_Thickness = 2 mm"
equation "PCB_Bottom_Z_Clearance = 3 mm"
equation "d85 = -PCB_Bottom_Z_Clearance"
equation "PCB_Horizontal_Clearance = 1 mm"
equation "d87 = PCB_Horizontal_Clearance"
equation "d88 = PCB_Horizontal_Clearance + Enclosure_Wall_Thickness"
equation "d89 = -Enclosure_Wall_Thickness"
equation "d95 = PCB_Bottom_Z_Clearance"
equation "Cutout_Clearance = 1 mm"
equation "d102 = Cutout_Clearance"
equation "USB_C_Plug_X_Size = 14 mm"
equation "USB_C_Plug_Y_Size = 10 mm"
equation "d107 = USB_C_Plug_X_Size"
equation "d108 = USB_C_Plug_Y_Size"
equation "d112 = d111"
equation "d113 = Enclosure_Wall_Thickness"
equation "d115 = Enclosure_Wall_Thickness"
equation "Battery_Ceiling_Clearance = 2 mm"
equation "d117 = -Battery_Ceiling_Clearance"
equation "d120 = Enclosure_Wall_Thickness"
equation "Antenna_Hole_Diameter = 8 mm"
equation "Antenna_PCB_Center_Z_Offset = 5.5 mm"
equation "d124 = Antenna_PCB_Center_Z_Offset + PCB_Z_Size"
equation "d126 = Antenna_Hole_Diameter"
equation "Enclosure_Bolt_Flange_Diameter = 6 mm"
equation "d129 = Enclosure_Bolt_Flange_Diameter"
equation "d130 = Enclosure_Bolt_Flange_Diameter"
equation "d131 = Enclosure_Bolt_Flange_Diameter * 2"
equation "d132 = d131"
equation "d133 = d131"
equation "d134 = d131"
equation "d137 = Enclosure_Bolt_Flange_Diameter / 2"
equation "d159 = Enclosure_Wall_Thickness"
equation "d160 = Enclosure_Chamfer"
equation "Enclosure_Chamfer = 1 mm"
equation "d162 = Enclosure_Chamfer"
